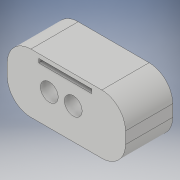
# Autodesk Inventor part: head
Saved by Autodesk Inventor 2019 (Build 230136000, 136)
## iProperties
Created: 2020-02-29
Part Number: head
Material: Generic
Document SubType Name: Modeling
Designer: Dell
Density: 1 g/cm^3
Appearance: Default
Author: Dell
Autodesk Inventor part; units mm, degrees
ref_plane "YZ Plane" through (0, 0, 0) normal (1, 0, 0) x (0, 1, 0)
ref_plane "XZ Plane" through (0, 0, 0) normal (0, 1, 0) x (-1, 0, 0)
ref_plane "XY Plane" through (0, 0, 0) normal (0, 0, 1) x (1, 0, 0)
sketch "Sketch1" plane through (0, 0, 0) normal (0, 0, 1) x (1, 0, 0)
  line L0 (20, 8.5409) -> (80, 8.5409)
  line L1 (100, -11.4591) -> (100, -21.4591)
  line L2 (80, -41.4591) -> (20, -41.4591)
  line L3 (0, -21.4591) -> (0, -11.4591)
  arc A0 (20, 8.5409) -> (0, -11.4591) centre (20, -11.4591) ccw
  arc A1 (100, -11.4591) -> (80, 8.5409) centre (80, -11.4591) ccw
  arc A2 (80, -41.4591) -> (100, -21.4591) centre (80, -21.4591) ccw
  arc A3 (0, -21.4591) -> (20, -41.4591) centre (20, -21.4591) ccw
  point P0 (0, 0)
  point P1 (100, -41.4591)
  point P2 (100, 8.5409)
  point P3 (0, -41.4591)
  dimension "d0" = 100
  dimension "d1" = 50
  dimension "d2" = 20
  constraints: 8 end point, 8 point on circle, 8 tangent, 6 point on line, 4 centre point, 3 equal radius, 2 parallel, 1 horizontal, 1 perpendicular
  measures "d0" distance of point (100, -41.459) point (0, -41.459)
  measures "d1" distance of point (100, 8.541) point (100, -41.459)
  measures "d2" radius of A0
extrude "Extrusion1" add sketch "Sketch1" along normal blind 40
sketch "Sketch3" plane through (0, 0, 40) normal (0, 0, 1) x (1, 0, 0)
  line L0 (26.6816, 5.0495) -> (71.4417, 5.0495)
  line L1 (71.4417, 5.0495) -> (71.4417, 1.6832)
  line L2 (71.4417, 1.6832) -> (26.6816, 1.6832)
  line L3 (26.6816, 1.6832) -> (26.6816, 5.0495)
  point P0 (0, 0)
  constraints: 8 end point, 2 parallel, 1 horizontal, 1 perpendicular
extrude "Extrusion2" cut sketch "Sketch3" against normal blind 40
sketch "Sketch4" plane through (0, 0, 40) normal (0, 0, 1) x (1, 0, 0)
  circle A0 centre (35.5822, -15.1611) radius 7.5
  circle A1 centre (55.8486, -15.1611) radius 7.5
  point P0 (0, 0)
  dimension "d16" = 15
  dimension "d17" = 15
  constraints: 2 centre point
  measures "d16" diameter of A0
  measures "d17" diameter of A1
hole "Hole2" at (35.5822, -15.1611, 40) at (55.8486, -15.1611, 40) direction (0, 0, -1) diameter 15 end through all
body "Solid1"
